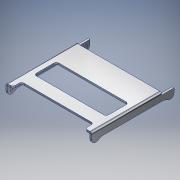
# Autodesk Inventor part: コックピット_サブフレーム_1_8
Saved by Autodesk Inventor 2018 (Build 220112000, 112)
## iProperties
Created: 2016-06-06
Part Number: コックピット_サブフレーム_1_8
Material: アルミニウム 5052
Document SubType Name: シート メタル
Designer: hiroaki
Density: 2.68 g/cm^3
Flat Pattern Width: 6.6 cm
Flat Pattern Length: 8.20736 cm
Flat Pattern Area: 54.1686 cm^2
Sheet Metal Rule: Default_mm
Sheet Metal Width: 66.000 mm
Sheet Metal Length: 82.074 mm
Sheet Metal Area: 5416.855 mm^2
Appearance: アルミニウム - フラット
Author: hiroaki
Autodesk Inventor part; units mm, degrees
ref_plane "YZ Plane" through (0, 0, 0) normal (1, 0, 0) x (0, 1, 0)
ref_plane "XZ Plane" through (0, 0, 0) normal (0, 1, 0) x (-1, 0, 0)
ref_plane "XY Plane" through (0, 0, 0) normal (0, 0, 1) x (1, 0, 0)
sketch "スケッチ1" plane through (0, 0, 0) normal (0, 0, 1) x (1, 0, 0)
  line L0 (-33, 33) -> (0, 33)
  line L1 (0, 33) -> (0, -33)
  line L2 (0, -33) -> (-33, -33)
  line L3 (-33, -33) -> (-33, 33)
  line L4 (-33, 30) -> (0, 30) construction
  line L5 (-33, -30) -> (0, -30) construction
  line L6 (-33, 0) -> (0, 0) construction
  dimension "d15" = 60
  dimension "d17" = 3
  dimension "d18" = 33
  constraints: 14 end point, 4 point on line, 3 perpendicular, 2 horizontal, 2 midpoint, 2 parallel, 1 coincident, 1 other
  measures "d15" distance between parallel lines of L5 L4
  measures "d17" distance between parallel lines of L4 L0
  measures "d18" distance of L0.start L0.end
extrude "押し出し1" add sketch "スケッチ1" along normal blind 1.5
sketch "スケッチ2" plane through (-33.0001, 33, -0.0001) normal (-1, 0, 0) x (0, -1, 0)
  line L0 (66, 0) -> (0, 0)
  line L1 (0, 0) -> (0, -6.9999)
  line L2 (0, -6.9999) -> (66, -6.9999)
  line L3 (66, -6.9999) -> (66, 0)
  constraints: 6 end point, 1 horizontal, 1 perpendicular, 1 vertical
edge flange "フランジ1" height 7 angle 90 thickness 1.5 bend radius 0.0001 thickness toward (-1, 0, 0) relief straight relief width 1.5 relief depth 0.75 edges at (-33, 0, 0) wall of the first edge with corners at (-33.0001, -33, -0.0001) (-33.0001, 33, -0.0001) (-33.0001, 33, -7) (-33.0001, -33, -7)
bend "曲げ1"
corner "コーナー1"
sketch "スケッチ3" plane through (-34.5001, -33, -7) normal (-1, 0, 0) x (0, 0, 1)
  line L0 (6.9999, 0) -> (6.9999, 66) projected
  line L1 (0, 66) -> (6.9999, 66) projected
  line L2 (0, 0) -> (0, 66) projected
  circle A0 centre (3, 63) radius 1.2
  circle A1 centre (3, 3) radius 1.2
  line L3 (7, 33) -> (0, 33) construction
  circle A2 centre (3, 63) radius 3 construction
  line L4 (3, 72.1771) -> (-13.2202, 72.1771)
  line L5 (-13.2202, 72.1771) -> (-13.2202, -4.077)
  line L6 (-13.2202, -4.077) -> (3, -4.077)
  line L7 (3, -4.077) -> (3, 0)
  line L8 (3, 72.1771) -> (3, 66)
  arc A3 (3, 66) -> (0.2751, 61.745) centre (3, 63) ccw
  line L9 (0.2751, 61.745) -> (1.9999, 58)
  line L10 (1.9999, 58) -> (1.9999, 8)
  line L11 (1.9999, 8) -> (0.2751, 4.255)
  arc A4 (0.2751, 4.255) -> (3, 0) centre (3, 3) ccw
  dimension "d48" = 2.4
  dimension "d49" = 60
  dimension "d50" = 3
  dimension "d52" = 50
  dimension "d55" = 5
  constraints: 18 end point, 5 centre point, 4 point on circle, 4 tangent, 3 coincident, 3 perpendicular, 3 vertical alignment, 2 equal radius, 2 symmetric about line, 2 vertical, 1 horizontal, 1 midpoint
  measures "d48" diameter of A0
  measures "d49" distance of A1.centre A0.centre
  measures "d50" distance from line of L2 A0.centre
  measures "d52" distance of L9.end L10.end
  measures "d55" distance between parallel lines of L0 L10
extrude "押し出し2" cut sketch "スケッチ3" against normal blind 2
mirror "ミラー1" about plane through (0, 0, 0) normal (1, 0, 0) of "押し出し2", "フランジ1", "押し出し1"
sketch "スケッチ4" plane through (0, 0, 1.5) normal (0, 0, 1) x (1, 0, 0)
  line L0 (-33, 33) -> (33, 33) projected
  line L1 (41.5665, 39.266) -> (-42.4114, 39.266)
  line L2 (-42.4114, 39.266) -> (-42.4114, 23)
  line L3 (-42.4114, 23) -> (41.5665, 23)
  line L4 (41.5665, 23) -> (41.5665, 39.266)
  point P0 (0, 0)
  dimension "d56" = 10
  constraints: 8 end point, 2 parallel, 1 horizontal, 1 perpendicular
  measures "d56" distance between parallel lines of L3 L0
extrude "押し出し3" cut sketch "スケッチ4" against normal blind 2
sketch "スケッチ5" plane through (0, 0, 1.5) normal (0, 0, 1) x (1, 0, 0)
  line L0 (-33, 23) -> (-33, -33) projected
  line L1 (-33, -33) -> (33, -33) projected
  line L2 (33, 23) -> (33, -33) projected
  line L3 (-29, 2) -> (29, 2)
  line L4 (29, 2) -> (29, -16)
  line L5 (29, -16) -> (-29, -16)
  line L6 (-29, -16) -> (-29, 2)
  line L7 (-29, -44) -> (29, -44)
  line L8 (29, -44) -> (29, -26)
  line L9 (29, -26) -> (-29, -26)
  line L10 (-29, -26) -> (-29, -44)
  point P0 (0, 0)
  dimension "d59" = 4
  dimension "d60" = 4
  dimension "d61" = 11
  dimension "d62" = 18
  dimension "d63" = 17
  constraints: 16 end point, 4 parallel, 2 horizontal, 2 perpendicular, 2 vertical alignment, 1 collinear
  measures "d59" distance between parallel lines of L0 L6
  measures "d60" distance between parallel lines of L2 L4
  measures "d61" distance between parallel lines of L1 L7
  measures "d62" distance of L9.end L7.start
  measures "d63" distance between parallel lines of L5 L1
extrude "押し出し4" cut sketch "スケッチ5" against normal blind 2
fillet "フィレット1" radius 2 8 edges at (29, 2, 0.75) (29, -16, 0.75) (-29, -16, 0.75) (-29, 2, 0.75) (-29, -26, 0.75) (29, -26, 0.75) (-29, -33, 0.75) (29, -33, 0.75)
sketch "スケッチ6" plane through (-34.5001, -25, -5.0001) normal (-1, 0, 0) x (0, 0, 1)
  circle A0 centre (1.0001, 55) radius 1.2 projected
  circle A1 centre (1.0001, 55) radius 1.2
  circle A2 centre (1.0001, -5) radius 1.2 projected
  circle A3 centre (1.0001, -5) radius 1.2
  point P0 (5.0001, 25)
  constraints: 2 centre point, 2 coincident
ref_plane "作業平面1" through (-32.9999, -53, -113) normal (-1, 0, 0) x (0, 0, 1)
extrude "押し出し5" add sketch "スケッチ6" against normal up to surface (1.5002 mm away)
sketch "スケッチ7" plane through (-33, 23, 1.5) normal (0, 1, 0) x (1, 0, 0)
  point P0 (33, 1.5)
sketch "スケッチ8" plane through (34.5001, -25, -5.0001) normal (1, 0, 0) x (0, 0, -1)
  circle A0 centre (-1.0001, 55) radius 1.2 projected
  circle A1 centre (-1.0001, 55) radius 1.2
  circle A2 centre (-1.0001, -5) radius 1.2 projected
  circle A3 centre (-1.0001, -5) radius 1.2
  point P0 (-5.0001, 25)
  constraints: 2 centre point, 2 coincident
ref_plane "作業平面2" through (33.0001, -53, -113) normal (1, 0, 0) x (0, 1, 0)
extrude "押し出し6" add sketch "スケッチ8" against normal up to surface (1.5 mm away)
equation "\"d15\" = d37"
equation "\"d49\" = d37"
equation "\"d60\" = d59"
equation "\"d38\" = BendReliefWidth"
equation "\"d39\" = BendReliefDepth"
equation "\"d40\" = MinimumRemnant"
equation "\"d41\" = BendRadius"
equation "\"d45\" = CornerReliefSize"
equation "\"d46\" = GapSize"
equation "\"d47\" = JacobiRadiusSize"
equation "\"d67\" = Thickness"
equation "\"BendRadius\" = Thickness"
equation "\"BendReliefWidth\" = Thickness"
equation "\"BendReliefDepth\" = 0.5 * Thickness"
equation "\"CornerReliefSize\" = 4 * Thickness"
equation "\"MinimumRemnant\" = 2 * Thickness"
equation "\"TransitionRadius\" = BendRadius"
equation "\"JacobiRadiusSize\" = BendRadius"
equation "\"GapSize\" = Thickness"
equation "\"d37\" = 60"
equation "\"Thickness\" = 1.5"
